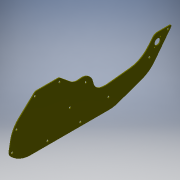
# Autodesk Inventor part: Cote_Droit
Saved by Autodesk Inventor 2016 (Build 200138000, 138)
## iProperties
Created: 2016-01-21
Part Number: Cote_Droit
Material: Fibre de verre - FR4
Document SubType Name: Modeling
Designer: sd
Density: 1.85 g/cm^3
Appearance: Générique
Mass: 50.8942 g
Surface Area: 358.439 cm^2
Volume: 27.5104 cm^3
Author: sd
Autodesk Inventor part; units mm, degrees
ref_plane "YZ Plane" through (0, 0, 0) normal (1, 0, 0) x (0, 1, 0)
ref_plane "XZ Plane" through (0, 0, 0) normal (0, 1, 0) x (-1, 0, 0)
ref_plane "XY Plane" through (0, 0, 0) normal (0, 0, 1) x (1, 0, 0)
sketch "Esquisse1" plane through (0, 0, 0) normal (1, 0, 0) x (0, 1, 0)
  line L0 (-80, -0.3825) -> (90, -0.3825)
  line L1 (90, -0.3825) -> (155.7273, 23)
  line L2 (155.7273, 23) -> (198, 78)
  line L3 (-80, -0.3825) -> (-102, 18)
  line L4 (-102, 18) -> (-95, 57)
  line L5 (-95, 57) -> (-53, 96)
  line L6 (-53, 96) -> (-9, 96)
  line L7 (-9, 96) -> (60.3686, 39.2438)
  line L8 (60.3686, 39.2438) -> (141.4545, 48)
  line L9 (141.4545, 48) -> (166, 78)
  line L10 (166, 78) -> (198, 78)
  point P0 (0, 0)
  dimension "d0" = 300
  dimension "d1" = 32
  dimension "d2" = 44
  dimension "d3" = 170
  constraints: 22 end point, 2 parallel, 1 horizontal, 1 perpendicular
  measures "d0" horizontal distance of L2.end L3.end
  measures "d1" distance of L9.end L2.end
  measures "d2" distance of L5.end L6.end
  measures "d3" distance of L0.start L0.end
extrude "Extrusion1" add sketch "Esquisse1" along normal blind 1.6
fillet "Congé1" radius 50 6 edges at (0.8, -95, 57) (0.8, -80, -0.3825) (0.8, 60.3686, 39.2438) (0.8, 141.4545, 48) (0.8, 155.7273, 23) (0.8, 90, -0.3825)
fillet "Congé2" radius 10 1 edges at (0.8, -102, 18)
fillet "Congé3" radius 10 1 edges at (0.8, 166, 78)
fillet "Congé4" radius 2 1 edges at (0.8, 198, 78)
fillet "Congé5" radius 5 2 edges at (0.8, -9, 96) (0.8, -53, 96)
sketch "Esquisse2" plane through (1.6, 0, 0) normal (1, 0, 0) x (0, 0, -1)
  line L0 (-94.664, -54.4388) -> (-68.3658, -82.7599) projected
  arc A0 (-23.7165, -100.974) -> (-14.2761, -97.5432) centre (-21.9498, -91.1313) ccw projected
  line L1 (-14.2761, -97.5432) -> (-11.2486, -93.92) projected
  line L2 (0.3825, -61.8602) -> (0.3825, 81.3711) projected
  line L3 (-34.6945, 164.7156) -> (-74.7812, 195.5261) projected
  line L4 (-78, 193.9403) -> (-78, 170.7388) projected
  line L5 (-52.5054, 44.1601) -> (-94.8698, -7.6186) projected
  circle A1 centre (-89.1175, -53.974) radius 2
  circle A2 centre (-19.9498, -95.7558) radius 2
  circle A3 centre (-6.6175, -30.7558) radius 2
  circle A4 centre (-39, 10.1327) radius 2
  circle A5 centre (-20.5549, 80.7442) radius 2
  circle A6 centre (-45.9957, 155.7442) radius 2
  circle A7 centre (-6.6175, 29.2442) radius 2
  circle A8 centre (-74, 189.8806) radius 2
  line L6 (-40.5594, -97.9509) -> (-23.7165, -100.974) projected
  circle A9 centre (-52.9562, -87.598) radius 2
  circle A10 centre (-89.1175, -8.974) radius 2
  line L7 (-96, -10.7848) -> (-96, -51.0365) projected
  point P0 (-41.4923, 81.1901)
  point P1 (0, 0)
  dimension "d11" = 4
  dimension "d13" = 4
  dimension "d14" = 4
  dimension "d15" = 4
  dimension "d16" = 4
  dimension "d17" = 4
  dimension "d22" = 2
  dimension "d23" = 5.5
  dimension "d24" = 7
  dimension "d25" = 4
  dimension "d26" = 7
  dimension "d27" = 60
  dimension "d28" = 65
  dimension "d31" = 41.8748
  dimension "d32" = 20.9374
  dimension "d36" = 14
  dimension "d37" = 75
  dimension "d38" = 4
  dimension "d39" = 4
  dimension "d40" = 4
  dimension "d43" = 4
  dimension "d44" = 8
  dimension "d45" = 8
  dimension "d64" = 4
  dimension "d65" = 45
  dimension "d66" = 89.5
  dimension "d67" = 89.5
  dimension "d68" = 47
  dimension "d70" = 32
  dimension "d71" = 57
  dimension "d72" = 51.5
  constraints: 10 centre point
  measures "d11" diameter of A1
  measures "d13" diameter of A4
  measures "d14" diameter of A2
  measures "d15" diameter of A3
  measures "d16" diameter of A5
  measures "d17" diameter of A6
  measures "d22" horizontal distance of A0.centre A2.centre
  measures "d23" distance from line of L1 A2.centre
  measures "d24" distance from line of L2 A3.centre
  measures "d25" diameter of A7
  measures "d26" distance from line of L2 A7.centre
  measures "d27" distance of A3.centre A7.centre
  measures "d28" vertical distance of A2.centre A3.centre
  measures "d31" horizontal distance of point (-41.492, 81.19) L2.end
  measures "d32" horizontal distance of L2.end A5.centre
  measures "d36" distance from line of L3 A6.centre
  measures "d37" vertical distance of A5.centre A6.centre
  measures "d38" diameter of A8
  measures "d39" distance from line of L3 A8.centre
  measures "d40" distance from line of L4 A8.centre
  measures "d43" diameter of A9
  measures "d44" distance from line of A9.centre L0
  measures "d45" distance from line of A9.centre L6
  measures "d64" diameter of A10
  measures "d65" distance of A10.centre A1.centre
  measures "d66" distance from line of L2 A1.centre
  measures "d67" distance from line of L2 A10.centre
  measures "d68" vertical distance of L6.end A1.centre
  measures "d70" distance from line of L5 A4.centre
  measures "d71" distance from line of L7 A4.centre
  measures "d72" vertical distance of A5.centre A7.centre
extrude "Extrusion2" cut sketch "Esquisse2" against normal blind 4
sketch "Esquisse3" plane through (1.6, 0, 0) normal (1, 0, 0) x (0, 0, -1)
  line L0 (-34.6945, 164.7156) -> (-74.7812, 195.5261) projected
  line L1 (-74.3324, 162.9992) -> (-63.8504, 154.423) projected
  circle A0 centre (-63.2102, 170.4635) radius 5.5
  line L2 (-52.7212, 161.1908) -> (-63.2102, 170.4635)
  line L3 (-63.2102, 170.4635) -> (-73.6991, 179.7361)
  circle A1 centre (-69.2039, 175.7621) radius 1.25
  circle A2 centre (-57.2165, 165.1648) radius 1.25
  point P0 (0, 0)
  dimension "d46" = 11
  dimension "d47" = 12.82
  dimension "d48" = 12.82
  dimension "d50" = 28
  dimension "d51" = 14
  dimension "d52" = 2.5
  dimension "d53" = 2.5
  dimension "d54" = 8
  dimension "d55" = 8
  dimension "d56" = 11.8599
  constraints: 4 end point, 3 centre point, 2 point on line, 1 collinear
  measures "d46" diameter of A0
  measures "d47" distance from line of L0 L2.end
  measures "d48" distance from line of L1 L2.end
  measures "d50" distance of L2.start L3.end
  measures "d51" distance of L2.end L3.end
  measures "d52" diameter of A1
  measures "d53" diameter of A2
  measures "d54" distance of L2.end A1.centre
  measures "d55" distance of L2.end A2.centre
  measures "d56" distance from line of L0 L3.end
extrude "Extrusion3" cut sketch "Esquisse3" against normal through all
sketch "Esquisse5" plane through (1.6, 0, 0) normal (1, 0, 0) x (0, 0, -1)
  circle A0 centre (-20.5549, 80.7442) radius 2 projected
  line L0 (-52.5054, 44.1601) -> (-94.8698, -7.6186) projected
  arc A1 (-47.0739, 50.7986) -> (-71.5553, 20.8768) centre (-55.3427, 32.5879) ccw
  line L1 (-47.0739, 50.7986) -> (-71.5553, 20.8768)
  point P0 (-96, -10.7848)
  point P1 (0, 0)
  dimension "d79" = 40
  dimension "d80" = 40
  dimension "d81" = 20
  constraints: 2 end point, 2 point on circle, 2 point on line, 1 centre point, 1 collinear
  measures "d79" distance of point (-96, -10.785) L1.end
  measures "d80" distance of A0.centre L1.start
  measures "d81" radius of A1
extrude "Extrusion5" add sketch "Esquisse5" against normal blind 1.6 contours L0 A1 L1
fillet "Congé7" radius 20 2 edges at (0.8, 20.8768, 71.5553) (0.8, 51.09, 47.7484)
sketch "Esquisse6" plane through (1.6, 0, 0) normal (1, 0, 0) x (0, 0, -1)
  line L0 (0.3825, -61.8602) -> (0.3825, 81.3711) projected
  circle A0 centre (-19.9498, -95.7558) radius 2 projected
  circle A1 centre (-64.6175, 39.2442) radius 2
  point P0 (0, 0)
  dimension "d85" = 4
  dimension "d86" = 65
  dimension "d87" = 135
  constraints: 1 centre point
  measures "d85" diameter of A1
  measures "d86" distance from line of L0 A1.centre
  measures "d87" vertical distance of A0.centre A1.centre
extrude "Extrusion6" cut sketch "Esquisse6" against normal through all contours A1
equation "\"d13\" = d11"
equation "\"d14\" = d11"
equation "\"d15\" = d11"
equation "\"d16\" = d11"
equation "\"d17\" = d11"
equation "\"d25\" = d11"
equation "\"d26\" = d24"
equation "\"d32\" = 0.5 * d31"
equation "\"d38\" = d11"
equation "\"d43\" = d11"
equation "\"d64\" = d11"
equation "\"d67\" = d66"
equation "\"d41\" = d43"
equation "\"d47\" = d48"
equation "\"d51\" = 0.5 * d50"
equation "\"d53\" = d52"
equation "\"d55\" = d54"
